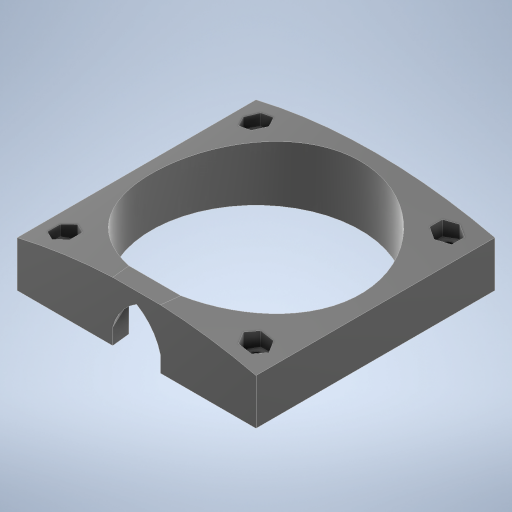
# Autodesk Inventor part: antenna_socket
Saved by Autodesk Inventor 2023 (Build 270158000, 158)
## iProperties
Created: 2023-06-06
Part Number: antenna_socket
Material: Acetal Resin, Black
Document SubType Name: Modeling
Designer: 310611102
Density: 1.425 g/cm^3
Appearance: Smooth - Black
Author: 310611102
Autodesk Inventor part; units mm, degrees
ref_plane "YZ Plane" through (0, 0, 0) normal (1, 0, 0) x (0, 1, 0)
ref_plane "XY Plane" through (0, 0, 0) normal (0, 0, 1) x (1, 0, 0)
sketch "Sketch1" plane through (0, 0, 0) normal (0, 0, 1) x (1, 0, 0)
  line L0 (-30, 7.5) -> (30, 7.5)
  line L1 (30, 7.5) -> (30, -7.5)
  line L2 (30, -7.5) -> (-30, -7.5)
  line L3 (-30, -7.5) -> (-30, 7.5)
  line L4 (-30, 7.5) -> (30, -7.5) construction
  line L5 (30, 7.5) -> (-30, -7.5) construction
  point P0 (0, 0)
  dimension "d0" = 60
  dimension "d1" = 15
  constraints: 12 end point, 2 midpoint, 2 parallel, 1 horizontal, 1 perpendicular
  measures "d0" distance of L0.start L0.end
  measures "d1" distance of L0.end L1.end
extrude "Extrusion1" add sketch "Sketch1" along normal blind 60
sketch "Sketch3" plane through (-30, 7.5, 0) normal (0, 1, 0) x (1, 0, 0)
  circle A0 centre (30, -30) radius 26.25
  line L0 (60, 0) -> (0, 0) projected
  line L1 (60, -60) -> (0, -60) projected
  line L2 (60, 0) -> (60, -60) projected
  line L3 (36.5, -55.4325) -> (36, -60)
  line L4 (36, -60) -> (24, -60)
  line L5 (24, -60) -> (23.5, -55.4325)
  point P0 (30, 0)
  point P1 (31.6579, -56.1976)
  point P2 (30, 0)
  point P3 (60, -30)
  point P4 (30, -60)
  point P5 (24, -60)
  dimension "d14" = 52.5
  dimension "d16" = 30
  dimension "d17" = 12
  dimension "d18" = 13
  dimension "d26" = 25.4325
  constraints: 6 end point, 3 midpoint, 3 point on circle, 2 vertical alignment, 1 centre point, 1 equal length, 1 horizontal, 1 horizontal alignment
  measures "d14" diameter of A0
  measures "d16" distance from line of A0.centre L4
  measures "d17" distance of L3.end L4.end
  measures "d18" distance of L3.start L5.end
  measures "d26" vertical distance of L3.start A0.centre
extrude "Extrusion3" cut sketch "Sketch3" against normal blind 15
sketch "Sketch4" plane through (0, 0, 60) normal (0, 0, 1) x (1, 0, 0)
  circle A0 centre (0, -122.5) radius 130
  line L0 (-26.25, 7.5) -> (26.25, 7.5) projected
  point P0 (0, 0)
  point P1 (-6.5, 7.5)
  point P2 (6.5, 7.5)
  dimension "d19" = 260
  constraints: 1 centre point, 1 tangent, 1 vertical alignment
  measures "d19" diameter of A0
extrude "Extrusion4" cut sketch "Sketch4" against normal through all keep common part
sketch "Sketch6" plane through (0, 0, 60) normal (0, 0, 1) x (1, 0, 0)
  arc A0 (0, 4.5) -> (-6, -3.5) centre (6.6, -6.7) ccw
  line L0 (0, 0) -> (0, -5.1929) construction
  arc A1 (6, -3.5) -> (0, 4.5) centre (-6.6, -6.7) ccw
  line L1 (-6, -3.5) -> (-6, 7.3615)
  line L2 (6, 7.3615) -> (6, -3.5)
  line L3 (-6, 7.3615) -> (6, 7.3615)
  line L4 (26.25, -7.5) -> (-26.25, -7.5) construction
  line L5 (-6, -7.5) -> (-6, 7.3615) construction
  point P0 (6.5, -7.5)
  point P1 (-6.5, -7.5)
  dimension "d27" = 13
  dimension "d31" = 12
  dimension "d35" = 4
  constraints: 8 end point, 4 point on circle, 2 centre point, 2 symmetric about line, 2 vertical, 1 point on line, 1 other
  measures "d27" radius of A0
  measures "d31" distance from line of L4 A0.start
  measures "d35" distance from line of L4 L1.start
ref_plane "Work Plane1" through (6.5, 7.3374, 55.4325) normal (0, 0, 1) x (1, 0, 0)
sketch "Sketch7" plane through (6.5, 7.3374, 55.4325) normal (0, 0, 1) x (1, 0, 0)
  line L0 (19.75, -14.8374) -> (-32.75, -14.8374) construction
  line L1 (-6.5, -14.8374) -> (-6.5, -0.6329) construction
  line L2 (-13, 0) -> (-13, -14.8374) construction
  line L3 (0, 0) -> (0, -14.8374) construction
  line L4 (-6.5, -14.8374) -> (-6.5, 0.8827) construction
  arc A0 (-6.5, -0.8374) -> (-13, -7.8374) centre (-0.8899, -12.5646) ccw
  arc A1 (0, -7.8374) -> (-6.5, -0.8374) centre (-12.1101, -12.5646) ccw
  line L5 (-13, 0) -> (0, 0)
  line L6 (-13, -7.8374) -> (-13, 0)
  line L7 (0, -7.8374) -> (0, 0)
  dimension "d32" = 14
  dimension "d33" = 13
  dimension "d34" = 7
  constraints: 10 end point, 4 point on circle, 3 point on line, 2 centre point, 2 symmetric about line, 2 vertical, 1 collinear, 1 horizontal, 1 midpoint, 1 other
  measures "d32" distance from line of L0 A0.start
  measures "d33" radius of A0
  measures "d34" distance from line of L0 L6.start
loft "Loft1" add profiles "Sketch7", "Sketch6"
ref_plane "Work Plane2" through (0, 7.5, 60) normal (0, 1, 0) x (-1, 0, 0)
sketch "Sketch8" plane through (0, 7.5, 60) normal (0, 1, 0) x (-1, 0, 0)
  line L0 (22.3834, -56.8) -> (20.7668, -54)
  line L1 (20.7668, -54) -> (22.3834, -51.2)
  line L2 (22.3834, -51.2) -> (25.6166, -51.2)
  line L3 (25.6166, -51.2) -> (27.2332, -54)
  line L4 (27.2332, -54) -> (25.6166, -56.8)
  line L5 (25.6166, -56.8) -> (22.3834, -56.8)
  arc A0 (-6.5, -4.5675) -> (6.5, -4.5675) centre (0, -30) ccw construction
  line L6 (26.8, -7.6166) -> (24, -9.2332)
  line L7 (24, -9.2332) -> (21.2, -7.6166)
  line L8 (21.2, -7.6166) -> (21.2, -4.3834)
  line L9 (21.2, -4.3834) -> (24, -2.7668)
  line L10 (24, -2.7668) -> (26.8, -4.3834)
  line L11 (26.8, -4.3834) -> (26.8, -7.6166)
  line L12 (-22.3834, -3.2) -> (-20.7668, -6)
  line L13 (-20.7668, -6) -> (-22.3834, -8.8)
  line L14 (-22.3834, -8.8) -> (-25.6166, -8.8)
  line L15 (-25.6166, -8.8) -> (-27.2332, -6)
  line L16 (-27.2332, -6) -> (-25.6166, -3.2)
  line L17 (-25.6166, -3.2) -> (-22.3834, -3.2)
  line L18 (-26.8, -52.3834) -> (-24, -50.7668)
  line L19 (-24, -50.7668) -> (-21.2, -52.3834)
  line L20 (-21.2, -52.3834) -> (-21.2, -55.6166)
  line L21 (-21.2, -55.6166) -> (-24, -57.2332)
  line L22 (-24, -57.2332) -> (-26.8, -55.6166)
  line L23 (-26.8, -55.6166) -> (-26.8, -52.3834)
  point P0 (0, -60)
  point P1 (24, -54)
  point P2 (24, -6)
  point P3 (-24, -6)
  point P4 (-24, -54)
  dimension "d40" = 24
  dimension "d41" = 5.6
  dimension "d42" = 24
  dimension "d45" = 360
  constraints: 48 end point, 1 coincident, 1 horizontal, 67 other
  measures "d40" horizontal distance of A0.centre point (24, -54)
  measures "d41" distance between parallel lines of L2 L5
  measures "d42" horizontal distance of A0.centre point (24, -54)
extrude "Extrusion5" cut sketch "Sketch8" against normal blind 5.5
sketch "Sketch9" plane through (0, 7.5, 60) normal (0, 1, 0) x (-1, 0, 0)
  circle A0 centre (24, -54) radius 1.65
  arc A1 (-6.5, -4.5675) -> (6.5, -4.5675) centre (0, -30) ccw construction
  circle A2 centre (24, -6) radius 1.65
  circle A3 centre (-24, -6) radius 1.65
  circle A4 centre (-24, -54) radius 1.65
  point P0 (0, -60)
  dimension "d49" = 3.3
  dimension "d50" = 24
  dimension "d51" = 24
  dimension "d54" = 360
  constraints: 4 centre point, 1 coincident, 10 other
  measures "d49" diameter of A0
  measures "d50" horizontal distance of A1.centre A0.centre
  measures "d51" horizontal distance of A1.centre A0.centre
extrude "Extrusion6" cut sketch "Sketch9" against normal through all
body "Solid1"
